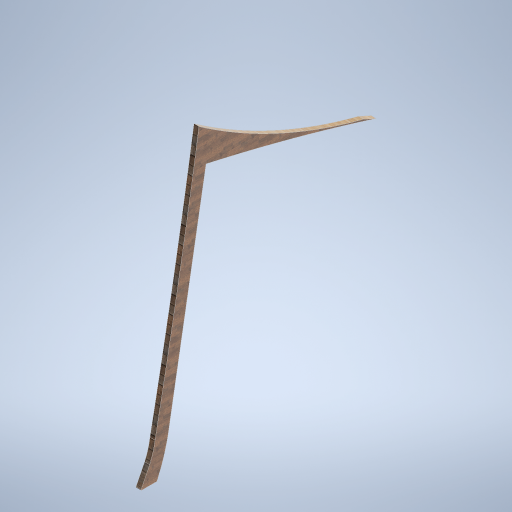
# Autodesk Inventor part: side_curve_beam_01
Saved by Autodesk Inventor 2024.2 (Build 282272000, 272)
## iProperties
Created: 2024-05-24
Part Number: side_curve_beam_01
Material: Wood (Maple)
Document SubType Name: Modeling
Designer: LOSTER_1
Density: 0.67 g/cm^3
Appearance: Natural Maple - Glossy Dark Tint
Author: LOSTER_1
Autodesk Inventor part; units mm, degrees
ref_plane "YZ Plane" through (0, 0, 0) normal (1, 0, 0) x (0, 1, 0)
ref_plane "XZ Plane" through (0, 0, 0) normal (0, 1, 0) x (-1, 0, 0)
ref_plane "XY Plane" through (0, 0, 0) normal (0, 0, 1) x (1, 0, 0)
sketch "Sketch1" plane through (0, 0, 0) normal (1, 0, 0) x (0, 1, 0)
  arc A0 (-3036.8928, 1718.534) -> (-4533.7659, -1525.4078) centre (5148.5741, -4025.866) ccw
  line L0 (-2952.6352, 1659.5361) -> (-2978.0832, 1677.355) construction
  arc A1 (-4650.0642, -1800.7835) -> (-4642.0762, -1823.7902) centre (-4600.2584, -1796.3809) ccw
  line L1 (-2978.0832, 1677.355) -> (-3036.8928, 1718.534)
  line L2 (-3036.8928, 1718.534) -> (-7960.9316, 2586.7748) construction
  line L3 (-3036.8928, 1718.534) -> (1963.1072, 1718.534) construction
  line L4 (-4650.0642, -1800.7835) -> (-4639.2556, -1760.4453) construction
  line L5 (-4650.0642, -1800.7835) -> (-1150.0642, -1800.7835) construction
  arc A2 (-8456.6899, 2457.4585) -> (-8005.9575, 2331.4201) centre (-7331.1025, 5613.7675) ccw
  arc A3 (-4533.4927, -1524.3501) -> (-4646.236, -1776.7324) centre (3169.9502, -5116.9769) ccw
  arc A4 (-2938.1875, 1679.4091) -> (-2952.6352, 1659.5361) centre (5142.9986, -4210.7887) ccw construction
  ellipse E0 centre (-3847.8838, -1113.1525) end of major axis (-3847.8838, -1913.1525) minor radius 800 (-4533.7659, -1524.936) -> (-4533.6807, -1525.0779) ccw
  ellipse E1 centre (-3847.8838, -1113.1525) end of major axis (-3847.8838, -1913.1525) minor radius 800 (-4256.7401, -1800.7835) -> (-4256.5248, -1800.9116) ccw
  line L6 (-8329.4706, 2692.6705) -> (-8685.4919, 2870.2518)
  line L7 (-8685.4919, 2870.2518) -> (-8685.4919, 2548.6634)
  line L8 (-8685.4919, 2548.6634) -> (-8456.6899, 2457.4585)
  arc A5 (-8329.4706, 2692.6705) -> (-7960.9316, 2586.7748) centre (-7766.0005, 3959.4195) ccw
  arc A6 (-7960.9316, 2586.7748) -> (-3036.8928, 1718.534) centre (15334.3466, 120303.9359) ccw
  arc A7 (-4645.5197, -1775.0569) -> (-3744.1975, 1579.9568) centre (-42788.682, 10270.6548) ccw
  line L9 (-8005.9575, 2331.4201) -> (-3744.1975, 1579.9568)
  point P0 (0, 0)
  dimension "d0" = 5000
  dimension "d1" = 170
  dimension "d4" = 75
  dimension "d9" = 120000
  dimension "d13" = 40000
  constraints: 20 end point, 20 point on circle, 8 centre point, 2 horizontal, 2 point on line, 1 equal length, 1 vertical, 8 other
  measures "d0" distance of L1.end L2.end
  measures "d1" angle of L3 L2
  measures "d4" angle of L5 L4
  measures "d9" radius of A6
  measures "d13" radius of A7
extrude "Extrusion2" add sketch "Sketch1" along normal blind 100 contours A0 A3 A7 L9 A2 L8 L7 L6 A5 A6
fillet "Fillet1" radius 10 1 edges at (50, -8685.4919, 2870.2518)
body "Solid2"
